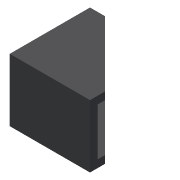
# Autodesk Inventor part: CornerBracket
Saved by Autodesk Inventor 2014 (Build 180170000, 170)
## iProperties
Created: 2014-08-11
Part Number: CornerBracket
Material: Generic
Document SubType Name: Modeling
Designer: Peele
Density: 1 g/cm^3
Appearance: Gray
Author: Peele
Autodesk Inventor part; units mm, degrees
ref_plane "YZ Plane" through (0, 0, 0) normal (1, 0, 0) x (0, 1, 0)
ref_plane "XZ Plane" through (0, 0, 0) normal (0, 1, 0) x (-1, 0, 0)
ref_plane "XY Plane" through (0, 0, 0) normal (0, 0, 1) x (1, 0, 0)
sketch "Sketch1" plane through (0, 0, 0) normal (0, 0, 1) x (1, 0, 0)
  line L0 (0, 0) -> (0, 32)
  line L1 (0, 32) -> (6, 32)
  line L2 (6, 32) -> (32, 6)
  line L3 (32, 6) -> (32, 0)
  line L4 (32, 0) -> (0, 0)
  dimension "d0" = 32
  dimension "d1" = 6
  constraints: 10 end point, 3 perpendicular, 2 parallel, 1 vertical
  measures "d0" distance of L0.start L0.end
  measures "d1" distance of L0.end L1.end
extrude "Extrusion1" add sketch "Sketch1" along normal mid plane 25
sketch "Sketch2" plane through (0, 32, 12.5) normal (0, 1, 0) x (1, 0, 0)
  line L0 (0, 0) -> (0, 25) projected
  line L1 (6, 0) -> (0, 0) projected
  line L2 (0, 25) -> (6, 25) projected
  line L3 (3, 22) -> (32, 22)
  line L4 (32, 22) -> (32, 3)
  line L5 (32, 3) -> (3, 3)
  line L6 (3, 3) -> (3, 22)
  line L7 (32, 0) -> (32, 25) projected
  point P0 (0, 12.5)
  dimension "d4" = 3
  dimension "d5" = 3
  dimension "d6" = 3
  constraints: 8 end point, 2 parallel, 1 collinear, 1 horizontal, 1 perpendicular
  measures "d4" distance between parallel lines of L2 L3
  measures "d5" distance between parallel lines of L5 L1
  measures "d6" distance between parallel lines of L0 L6
extrude "Extrusion2" cut sketch "Sketch2" against normal blind 29
equation "\"d5\" = d4"
equation "\"d6\" = d4"
body "Solid1"
